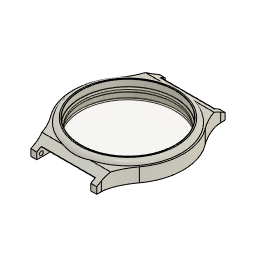
PersonalReminder_3Dmodel (Autodesk Fusion 360 archive; units mm, degrees)
design "CasioMq24"
Autodesk Fusion 360 part; units mm, degrees
sketch "CasioMq24SketchMainBody" plane through (0, 0, 0) normal (0, 0, 1) x (1, 0, 0)
  circle A0 centre (0, 0) radius 16.25
  circle A1 centre (0, 0) radius 14.4
  circle A2 centre (0, 0) radius 16.75
  line L0 (-10, 18.1) -> (0, 18.1)
  line L1 (0, 18.1) -> (0, 0) construction
  line L2 (0, 0) -> (16.75, 0) construction
  line L3 (0, 0) -> (-16.75, 0) construction
  spline S0 degree 5 poles (-10, 18.1) (-10, 17.8332) (-10.0336, 17.2821) (-10.1849, 16.4029) (-10.566, 15.1406) (-11.2795, 13.467) (-12.0233, 12.0871) (-12.6888, 11.0411) (-13.1848, 10.34) (-13.4459, 9.9886) knots 0 0 0 0 0 0 0.2 0.4 0.6 0.8 1 1 1 1 1 1
  line L4 (-10, 18.7) -> (-10, 17.5)
  line L5 (-12.8437, 10.7991) -> (-14.048, 9.178)
  spline S1 degree 5 poles (10, 18.1) (10, 17.8332) (10.0336, 17.2821) (10.1849, 16.4029) (10.566, 15.1406) (11.2795, 13.467) (12.0233, 12.0871) (12.6888, 11.0411) (13.1848, 10.34) (13.4459, 9.9886) knots 0 0 0 0 0 0 0.2 0.4 0.6 0.8 1 1 1 1 1 1
  line L6 (10, 18.7) -> (10, 17.5)
  line L7 (12.8437, 10.7991) -> (14.048, 9.178)
  line L8 (10, 18.1) -> (0, 18.1)
  spline S2 degree 5 poles (-10, -18.1) (-10, -17.8332) (-10.0336, -17.2821) (-10.1849, -16.4029) (-10.566, -15.1406) (-11.2795, -13.467) (-12.0233, -12.0871) (-12.6888, -11.0411) (-13.1848, -10.34) (-13.4459, -9.9886) knots 0 0 0 0 0 0 0.2 0.4 0.6 0.8 1 1 1 1 1 1
  line L9 (-10, -18.7) -> (-10, -17.5)
  line L10 (-12.8437, -10.7991) -> (-14.048, -9.178)
  line L11 (-10, -18.1) -> (0, -18.1)
  line L12 (10, -18.1) -> (0, -18.1)
  spline S3 degree 5 poles (10, -18.1) (10, -17.8332) (10.0336, -17.2821) (10.1849, -16.4029) (10.566, -15.1406) (11.2795, -13.467) (12.0233, -12.0871) (12.6888, -11.0411) (13.1848, -10.34) (13.4459, -9.9886) knots 0 0 0 0 0 0 0.2 0.4 0.6 0.8 1 1 1 1 1 1
  line L13 (10, -18.7) -> (10, -17.5)
  line L14 (12.8437, -10.7991) -> (14.048, -9.178)
  line L15 (16.75, 0) -> (19.15, 0) construction
  line L16 (17.95, 2.9) -> (17.95, -2.9)
  spline S4 degree 5 poles (15.3957, 6.5981) (15.4474, 6.4974) (15.5594, 6.2792) (15.7531, 5.9019) (16.0608, 5.3152) (16.536, 4.5058) (17.0134, 3.8459) (17.4477, 3.3649) (17.7761, 3.0534) (17.95, 2.9) knots 0 0 0 0 0 0 0.2 0.4 0.6 0.8 1 1 1 1 1 1
  line L17 (17.27, 3.5) -> (18.63, 2.3)
  line L18 (15.1914, 6.9963) -> (15.6, 6.2)
  line L19 (17.95, -2.9) -> (17.95, 2.9)
  spline S5 degree 5 poles (15.3957, -6.5981) (15.4474, -6.4974) (15.5594, -6.2792) (15.7531, -5.9019) (16.0608, -5.3152) (16.536, -4.5058) (17.0134, -3.8459) (17.4477, -3.3649) (17.7761, -3.0534) (17.95, -2.9) knots 0 0 0 0 0 0 0.2 0.4 0.6 0.8 1 1 1 1 1 1
  line L20 (15.1914, -6.9963) -> (15.6, -6.2)
  line L21 (17.27, -3.5) -> (18.63, -2.3)
  line L22 (-10, 15.25) -> (-6.9282, 15.25)
  spline S6 degree 5 poles (-10, 15.25) (-10.0308, 15.0847) (-10.1148, 14.7548) (-10.3082, 14.2626) (-10.6811, 13.6097) (-11.2659, 12.7894) (-11.7792, 12.1195) (-12.1718, 11.6033) (-12.4349, 11.2518) (-12.5668, 11.0743) knots 0 0 0 0 0 0 0.2 0.4 0.6 0.8 1 1 1 1 1 1
  line L23 (-9.9252, 15.6518) -> (-10.0748, 14.8482)
  line L24 (-12.2362, 11.5192) -> (-12.8973, 10.6293)
  line L25 (-10, 18.1) -> (10, 18.1)
  line L26 (10, 18.1) -> (10, 19.5)
  line L27 (10, 19.5) -> (-10, 19.5)
  line L28 (-10, 19.5) -> (-10, 18.1)
  line L29 (10, -19.5) -> (-10, -19.5)
  line L30 (-10, -19.5) -> (-10, -18.1)
  line L31 (10, -18.1) -> (10, -19.5)
  spline S7 degree 5 poles (10, 15.25) (10.0308, 15.0847) (10.1148, 14.7548) (10.3082, 14.2626) (10.6811, 13.6097) (11.2659, 12.7894) (11.7792, 12.1195) (12.1718, 11.6033) (12.4349, 11.2518) (12.5668, 11.0743) knots 0 0 0 0 0 0 0.2 0.4 0.6 0.8 1 1 1 1 1 1
  line L32 (9.9252, 15.6518) -> (10.0748, 14.8482)
  line L33 (12.2362, 11.5192) -> (12.8973, 10.6293)
  line L34 (10, 15.25) -> (6.9282, 15.25)
  line L35 (-10, -15.25) -> (-6.9282, -15.25)
  spline S8 degree 5 poles (-10, -15.25) (-10.0308, -15.0847) (-10.1148, -14.7548) (-10.3082, -14.2626) (-10.6811, -13.6097) (-11.2659, -12.7894) (-11.7792, -12.1195) (-12.1718, -11.6033) (-12.4349, -11.2518) (-12.5668, -11.0743) knots 0 0 0 0 0 0 0.2 0.4 0.6 0.8 1 1 1 1 1 1
  line L36 (-9.9252, -15.6518) -> (-10.0748, -14.8482)
  line L37 (-12.2362, -11.5192) -> (-12.8973, -10.6293)
  line L38 (10, -15.25) -> (6.9282, -15.25)
  spline S9 degree 5 poles (10, -15.25) (10.0308, -15.0847) (10.1148, -14.7548) (10.3082, -14.2626) (10.6811, -13.6097) (11.2659, -12.7894) (11.7792, -12.1195) (12.1718, -11.6033) (12.4349, -11.2518) (12.5668, -11.0743) knots 0 0 0 0 0 0 0.2 0.4 0.6 0.8 1 1 1 1 1 1
  line L39 (9.9252, -15.6518) -> (10.0748, -14.8482)
  line L40 (12.2362, -11.5192) -> (12.8973, -10.6293)
  line L41 (10, 18.1) -> (10, 13.4374) construction
  line L42 (-10, 18.1) -> (-10, 13.4374) construction
  line L43 (10, -18.1) -> (10, -13.4374) construction
  line L44 (-10, -18.1) -> (-10, -13.4374) construction
  line L45 (-6.9282, -15.25) -> (6.9282, -15.25)
  line L46 (-6.9282, 15.25) -> (6.9282, 15.25)
  line L47 (-8.2, 19.5) -> (8.2, 19.5)
  line L48 (8.2, 19.5) -> (8.2, 15.25)
  line L49 (8.2, 15.25) -> (-8.2, 15.25)
  line L50 (-8.2, 15.25) -> (-8.2, 19.5)
  line L51 (8.2, -19.5) -> (8.2, -15.25)
  line L52 (8.2, -15.25) -> (-8.2, -15.25)
  line L53 (-8.2, -15.25) -> (-8.2, -19.5)
  line L54 (-8.2, -19.5) -> (8.2, -19.5)
  circle A3 centre (0, 0) radius 13.9
  circle A4 centre (0, 0) radius 14.325
  dimension "d1" = 10
  dimension "d2" = 28.8
  dimension "d3" = 32.5
  dimension "d4" = 33.5
  dimension "d5" = 18.1
  dimension "d6" = 5.8
  dimension "d7" = 1.2
  dimension "d9" = 2.85
  dimension "d10" = 1.4
  dimension "d62" = 1.8
  dimension "d63" = 1.8
  dimension "d83" = -0.5
  dimension "d99" = 28.65
  constraint coincident A0.centre A1.centre
  constraint horizontal L0
  constraint perpendicular L0 L1
  constraint coincident A2 L2.end
  constraint horizontal L2
  constraint coincident A2 L3.end
  constraint parallel L2 L3
  constraint coincident A2 S0.end
  constraint midpoint L0.start L4
  constraint midpoint S0.end L5
  constraint tangent A2 L5
  constraint symmetric L0.start L1 S1.start
  constraint symmetric L0.end L1 L8.end
  constraint symmetric L1 S0.end S1.end
  constraint symmetric L1 L4.start L6.start
  constraint symmetric L1 L4.end L6.end
  constraint symmetric L1 L5.start L7.start
  constraint symmetric L1 L5.end L7.end
  constraint symmetric L0.start L2 S2.start
  constraint symmetric L0.end L2 L11.end
  constraint symmetric L2 S0.end S2.end
  constraint symmetric L2 L4.start L9.start
  constraint symmetric L2 L4.end L9.end
  constraint symmetric L2 L5.start L10.start
  constraint symmetric L2 L5.end L10.end
  constraint symmetric L2 S1.start L12.start
  constraint symmetric L2 S1.end S3.end
  constraint symmetric L2 L6.start L13.start
  constraint symmetric L2 L6.end L13.end
  constraint symmetric L2 L7.start L14.start
  constraint symmetric L2 L7.end L14.end
  constraint symmetric L2 L0.end L11.end
  constraint parallel L2 L15
  constraint perpendicular L15 L16
  constraint midpoint L15 L16
  constraint coincident A2 S4.start
  constraint midpoint L16.start L17
  constraint midpoint S4.start L18
  constraint symmetric L15 L16.start L16.end
  constraint symmetric L15 L16.end L16.start
  constraint symmetric L15 S4.start S5.start
  constraint symmetric L15 L17.start L21.start
  constraint symmetric L15 L17.end L21.end
  constraint symmetric L15 L18.start L20.start
  constraint symmetric L15 L18.end L20.end
  constraint coincident A2 L22.end
  constraint parallel L0 L22
  constraint coincident A2 S6.end
  constraint midpoint L22.start L23
  constraint midpoint S6.end L24
  constraint parallel L5 L24
  constraint horizontal L25
  constraint vertical L26
  constraint horizontal L27
  constraint vertical L28
  constraint symmetric L2 L26.end L29.start
  constraint symmetric L2 L27.end L29.end
  constraint symmetric L1 L22.start S7.start
  constraint symmetric L1 L22.end L34.end
  constraint symmetric L1 S6.end S7.end
  constraint symmetric L1 L23.start L32.start
  constraint symmetric L1 L23.end L32.end
  constraint symmetric L1 L24.start L33.start
  constraint symmetric L1 L24.end L33.end
  constraint symmetric L2 L22.start L35.start
  constraint symmetric L2 L22.end L35.end
  constraint symmetric L2 S6.end S8.end
  constraint symmetric L2 L23.start L36.start
  constraint symmetric L2 L23.end L36.end
  constraint symmetric L2 L24.start L37.start
  constraint symmetric L2 L24.end L37.end
  constraint symmetric L2 S7.start L38.start
  constraint symmetric L2 S7.end S9.end
  constraint symmetric L2 L32.start L39.start
  constraint symmetric L2 L32.end L39.end
  constraint symmetric L2 L33.start L40.start
  constraint symmetric L2 L33.end L40.end
  constraint symmetric L2 L34.end L38.end
  constraint coincident A2 L41.end
  constraint coincident A2 L42.end
  constraint coincident S7.start L41
  constraint coincident A2 L43.end
  constraint perpendicular L12 L43
  constraint coincident A2 L44.end
  constraint parallel L38 L45
  constraint symmetric L3 L35.end L22.end
  constraint symmetric L3 L38.end L34.end
  constraint horizontal L47
  constraint vertical L48
  constraint horizontal L49
  constraint vertical L50
  constraint coincident L34 L48.end
  constraint coincident L27 L47.start
  constraint symmetric L3 L47.start L53.end
  constraint symmetric L3 L47.end L51.start
  constraint symmetric L3 L48.end L51.end
  constraint symmetric L3 L49.end L52.end
  constraint coincident S1.start L26
  constraint concentric A2 A4
  measures "d1" distance of L0.start L0.end
  measures "d2" diameter of A1
  measures "d3" diameter of A0
  measures "d4" diameter of A2
  measures "d5" distance of L0.end A0.centre
  measures "d6" distance of L16.start L16.end
  measures "d7" distance of L2.end L16
  measures "d9" distance of L0 L22
  measures "d10" distance of L25 L27
  measures "d62" distance of L28 L50
  measures "d63" distance of L26 L48
  measures "d99" diameter of A4
extrude "Extrude18" add sketch "CasioMq24SketchMainBody" along normal blind 2 contours A3 | A4 makes body 1
extrude "Extrude1" add sketch "CasioMq24SketchMainBody" along normal blind 4.2 separate body contours A0 A2 L45 L46 L49 L52 | A0 A2 L46 L49 | A0 A2 L45 L52 | A0 A2 L45 L46 L49 L52 | A2 S7 L33 L34 L49 | A2 L0 L8 L22 L25 L34 L48 L49 L50 | A2 L11 L12 L35 L38 L51 L52 L53 | A2 L38 S9 L40 L52 | A2 L22 S6 L24 L49 | A2 S1 L8 L25 S7 L33 L34 L48 | A2 L35 S8 L37 L52 | A2 L12 S3 L38 S9 L40 L51 | A2 L0 S0 L22 S6 L24 L25 L50 | L6 L8 L25 L26 L27 L48 | A2 S2 L11 L35 S8 L37 L53 | L12 L13 L29 L31 L51 | L0 L4 L25 L27 L28 L50 | L9 L11 L29 L30 L53 makes body 2
extrude "Extrude2" add sketch "CasioMq24SketchMainBody" along normal blind 5.4 contours A0 L45 L46 L49 L52 | A0 L46 L49 | A0 L45 L52 bodies 2
chamfer "Chamfer1" distance 3.797 angle 30 3 edges at (9.1, -19.5, 4.2) (-9.1, -19.5, 4.2) (9.1, 19.5, 4.2) measured on face at (0.4048, -17.4682, 4.2) measured on face at (0.4048, -17.4682, 4.2) measured on face at (0.4048, -17.4682, 4.2) on bodies 2
fillet "Fillet1" radius 1.5 1 edges at (-15.1503, -5.8763, 5.4) on bodies 2
extrude "Extrude11" cut sketch "CasioMq24SketchMainBody" along normal blind 2.7 contours A0 L46 L49 | A0 A2 L46 L49 | A0 A2 L45 L52 | A0 L45 L52 | A2 L0 L8 L22 L25 L34 L48 L49 L50 | A2 L11 L12 L35 L38 L51 L52 L53 bodies 2
sketch "BandHoles" plane through (-8.2, 0, 0) normal (1, 0, 0) x (0, 1, 0)
  line L0 (-18.1, 2.8161) -> (-19.5, 2.0078)
  line L1 (-19.5, 2.0078) -> (-19.5, 0)
  line L2 (-19.5, 0) -> (-15.25, 0)
  line L3 (-15.25, 0) -> (-15.25, 2.7)
  line L4 (-15.25, 2.7) -> (-18.1, 2.7)
  circle A0 centre (-18.1, 1.0039) radius 0.6
  line L5 (-19.5, 1.0039) -> (-18.1, 1.0039) construction
  line L6 (-18.1, 1.0039) -> (-18.1, 2.7006) construction
  line L7 (-18.1, 2.7) -> (-18.1, 2.8161)
  dimension "d70" = 1.2
  constraint midpoint L1 L5.start
  constraint coincident A0.centre L5.end
  constraint perpendicular L5 L6
  constraint coincident L6.end L7
  constraint parallel L2 L5
  measures "d70" diameter of A0
extrude "Extrude1'" add sketch "BandHoles" against normal blind 1 separate body contours A0 makes body 3 in component "BandPinHoleCutter"
mirror "Mirror1" about plane through (0, 0, 0) normal (0, 1, 0) of bodies 3 makes body 4 in component "BandPinHoleCutter"
mirror "Mirror2" about plane through (0, 0, 0) normal (1, 0, 0) of bodies 4 3 makes body 5 at (8.5333, -17.503, 0.9442) makes body 6 at (8.5333, 17.503, 0.9442) in component "BandPinHoleCutter"
combine "Combine1" operation cut target body 2 tool bodies 3 4 5 6
extrude "Extrude15" add sketch "CasioMq24SketchMainBody" along normal blind 1.4 from surface at 2 contours A1 | A4 bodies 2
copy_body "Body->Comp1" bodies 2 removing the originals makes body 7 in component "MainCase"
chamfer "Chamfer1'" distance 0.4 angle 45 2 edges at (-12.9594, 5.0265, 3.4) (-12.9594, 5.0265, 2) on bodies 7 in component "MainCase"
chamfer "Chamfer2" distance 0.5 angle 45 1 edges at (-13.4255, 5.2073, 0) on bodies 7 in component "MainCase"
copy_body "Body->Comp2" bodies 1 removing the originals makes body 8 in component "Plexi"
move_body "Move1" bodies 8 to x (1, 0, 0) y (0, 1, 0) z (0, 0, 1) at (0, 0, 3.4) in component "Plexi"
copy_body "CopyPasteBodies1" bodies 8 makes body 9
move_body "Move2" bodies 9 to x (1, 0, 0) y (0, 1, 0) z (0, 0, 1) at (0, 0, -3.4)
copy_body "CutPasteBodies1" bodies 9 removing the originals makes body 10 in component "Plexi"
component "BandPinHoleCutter" placed x (1, 0, 0) y (0, 1, 0) z (0, 0, 1) at (0, 0, 0)
component "MainCase" placed x (1, 0, 0) y (0, 1, 0) z (0, 0, 1) at (0, 0, 0)
component "Plexi" placed x (1, 0, 0) y (0, 1, 0) z (0, 0, 1) at (0, 0, 0)
equation "d1 = ( 20 / 2 ) * 1 mm"
equation "d5 = ( ( 36.2 ) / 2 ) * 1 mm"
equation "d62 = d63"
equation "d87 = -0.5 mm - 0.2 mm"
equation "d89 = 0.35 mm"
equation "d90 = d89"
named bodies: "MainCase", "Plexi", "PlexiFront", "PlexiBack"
